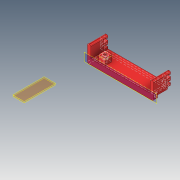
# Autodesk Inventor part: Prova A1
Saved by Autodesk Inventor 2019 (Build 230136000, 136)
## iProperties
Created: 2019-05-06
Part Number: Prova A1
Material: Generic
Document SubType Name: Modeling
Designer: giacomo
Density: 1 g/cm^3
Appearance: Light Red
Author: giacomo
Autodesk Inventor part; units mm, degrees
ref_plane "YZ Plane" through (0, 0, 0) normal (1, 0, 0) x (0, 1, 0)
ref_plane "XZ Plane" through (0, 0, 0) normal (0, 1, 0) x (-1, 0, 0)
ref_plane "XY Plane" through (0, 0, 0) normal (0, 0, 1) x (1, 0, 0)
sketch "Sketch1" plane through (0, 0, 0) normal (0, 1, 0) x (-1, 0, 0)
  line L0 (-50, 75) -> (50, 75)
  line L1 (50, 75) -> (50, -75)
  line L2 (50, -75) -> (-50, -75)
  line L3 (-50, -75) -> (-50, 75)
  line L4 (-50, 75) -> (50, -75) construction
  line L5 (50, 75) -> (-50, -75) construction
  point P0 (0, 0)
  dimension "d0" = 100
  dimension "d1" = 150
  constraints: 12 end point, 2 midpoint, 2 parallel, 1 horizontal, 1 perpendicular
  measures "d0" distance of L1.end L2.end
  measures "d1" distance of L0.end L1.end
extrude "Extrusion1" add sketch "Sketch1" along normal blind 8
sketch "Sketch3" plane through (0, 8, 0) normal (0, 1, 0) x (1, 0, 0)
  line L0 (-50, -75) -> (50, -75) projected
  line L1 (50, -75) -> (50, 75) projected
  line L2 (50, 75) -> (-50, 75) projected
  line L3 (-50, 75) -> (-50, -75) projected
  line L4 (45, 75) -> (45, -70)
  line L5 (-50, -75) -> (50, -75) projected
  line L6 (50, -75) -> (50, 75) projected
  line L7 (0, 0) -> (0, -83) construction
  line L8 (-45, 75) -> (-45, -70)
  line L9 (45, -70) -> (-45, -70)
  dimension "d4" = 5
  dimension "d5" = 5
  constraints: 8 end point, 3 parallel, 2 point on line, 1 perpendicular, 1 vertical, 1 other
  measures "d4" distance between parallel lines of L1 L4
  measures "d5" distance between parallel lines of L9 L0
extrude "Extrusion2" add sketch "Sketch3" along normal blind 18 contours L3 L2 L8 L9 L4 L1 L0
sketch "Sketch4" plane through (50, 0, -75) normal (0, 0, -1) x (-1, 0, 0)
  line L0 (100, 0) -> (0, 0) projected
  line L1 (100, 0) -> (100, 26) projected
  line L2 (95, 26) -> (100, 26) projected
  line L3 (95, 8) -> (95, 26) projected
  line L4 (5, 8) -> (95, 8) projected
  line L5 (5, 8) -> (5, 26) projected
  line L6 (0, 26) -> (5, 26) projected
  line L7 (0, 0) -> (0, 26) projected
  line L8 (95, 8) -> (5, 8) projected
  line L9 (5, 8) -> (5, 0)
  line L10 (95, 8) -> (95, 0)
  line L11 (0, 0) -> (100, 0) projected
  line L12 (0, 0) -> (0, 26) projected
  line L13 (5, 3) -> (95, 3)
  line L14 (5, 8) -> (95, 8) projected
  line L15 (5, 6) -> (95, 6)
  line L16 (5, 8) -> (0, 8)
  line L17 (100, 0) -> (0, 0) projected
  point P0 (50, 0)
  dimension "d8" = 3
  dimension "d9" = 3
  constraints: 10 end point, 8 point on line, 6 parallel, 2 perpendicular, 1 vertical
  measures "d8" distance between parallel lines of L0 L13
  measures "d9" distance between parallel lines of L13 L15
extrude "Extrusion3" add sketch "Sketch4" along normal blind 20 contours L0 L10 L3 L2 L1 | L0 L9 L13 L10 | L15 L9 L4 L10 | L7 L6 L5 L16
sketch "Sketch6" plane through (50, 0, 75) normal (1, 0, 0) x (0, 0, -1)
  line L0 (150, 0) -> (150, 8)
  line L1 (170, 26) -> (170, 8)
  line L2 (0, 0) -> (0, 26) projected
  line L3 (150, 8) -> (170, 8)
  line L4 (170, 26) -> (170, 8) projected
  line L5 (170, 11.2) -> (163, 9.7)
  line L6 (163, 9.7) -> (163, 15.7)
  line L7 (163, 15.7) -> (170, 14.2)
  line L8 (170, 19.3) -> (163, 17.8)
  line L9 (163, 17.8) -> (163, 23.8)
  line L10 (163, 23.8) -> (170, 22.3)
  line L11 (170, 22.3) -> (170, 19.3)
  line L12 (170, 14.2) -> (170, 11.2)
  point P0 (75, 0)
  dimension "d14" = 3
  dimension "d15" = 7
  dimension "d16" = 1.5
  dimension "d17" = 1.5
  dimension "d18" = 3
  dimension "d19" = 1.5
  dimension "d20" = 1.5
  dimension "d21" = 5.1
  dimension "d22" = 7
  dimension "d36" = 1.7
  constraints: 22 end point, 2 point on line, 2 vertical, 1 collinear, 1 horizontal, 1 parallel
  measures "d14" distance of L5.start L7.end
  measures "d15" distance between parallel lines of L1 L6
  measures "d16" vertical distance of L5.end L5.start
  measures "d17" vertical distance of L6.end L7.end
  measures "d18" distance of L8.start L10.end
  measures "d19" vertical distance of L8.end L8.start
  measures "d20" vertical distance of L10.start L10.end
  measures "d21" distance of L7.end L8.start
  measures "d22" distance between parallel lines of L4 L9
  measures "d36" distance from line of L3 L5.end
extrude "Extrusion4" cut sketch "Sketch6" against normal through all
fillet "Fillet1" radius 2 11 edges at (50, 0, 0) (50, 26, -10) (50, 13, 75) (0, 26, 75) (0, 0, 75) (-50, 26, -10) (-50, 13, 75) (-50, 0, -10) (45, 26, -12.5) (-45, 26, -12.5) (0, 26, 70)
sketch "Sketch11" plane through (-50, 9.7, -88) normal (-1, 0, 0) x (0, 0, 1)
  line L0 (9, 17.5) -> (0, 19.5) projected
  line L1 (0, 19.5) -> (0, 11.5) projected
  line L2 (0, 11.5) -> (9, 14) projected
  line L3 (9, 17.5) -> (9, 14) projected
  line L4 (9, 6) -> (0, 8.5) projected
  line L5 (0, 0) -> (9, 2.5) projected
  line L6 (0, 6) -> (0, 0) projected
  line L7 (9, 6) -> (9, 2.5) projected
  point P0 (88, -9.7)
sketch "Sketch12" plane through (-50, 2, 73) normal (-1, 0, 0) x (0, 0, 1)
  line L0 (-168, 28) -> (-168, 20)
  line L1 (-159, 26) -> (-168, 28)
  line L2 (-159, 26) -> (-159, 22.5)
  line L3 (-168, 20) -> (-159, 22.5)
  line L4 (-168, 17) -> (-168, 8.5)
  line L5 (-159, 14.5) -> (-168, 17)
  line L6 (-159, 14.5) -> (-159, 11)
  line L7 (-168, 8.5) -> (-159, 11)
  line L8 (-168, 0) -> (-168, 22) projected
  line L9 (-161, 19.2) -> (-161, 27.2) projected
  line L10 (-161, 27.2) -> (-168, 27.2)
  line L11 (-168, 22) -> (-168, 6) projected
  line L12 (-159, 17) -> (-168, 17)
  point P0 (-73, -2)
  constraints: 20 end point, 2 perpendicular, 2 point on line
sketch "Sketch15" plane through (45, 6, -75) normal (1, 0, 0) x (0, 0, -1)
  line L0 (0, 0) -> (0, 2) projected
  line L1 (0, 0) -> (20, 0) projected
  line L2 (20, 2) -> (20, 0) projected
  line L3 (0, 2) -> (20, 2) projected
  point P0 (-75, -6)
extrude "Extrusion8" add sketch "Sketch15" along normal blind 2.5
sketch "Sketch16" plane through (0, 8, 0) normal (0, 1, 0) x (1, 0, 0)
  line L0 (-45, -35) -> (-37, -35)
  line L1 (-37, -35) -> (-37, -15)
  line L2 (-37, -15) -> (-45, -15)
  line L3 (-45, -15) -> (-45, -35)
  line L4 (45, -70) -> (-45, -70) projected
  line L5 (-45, -70) -> (-45, 95) projected
  line L6 (32, -70) -> (45, -70)
  line L7 (45, -70) -> (45, -45)
  line L8 (45, -45) -> (32, -45)
  line L9 (32, -45) -> (32, -70)
  line L10 (45, 95) -> (45, -70) projected
  point P0 (0, 0)
  dimension "d39" = 35
  dimension "d40" = 0
  dimension "d41" = 8
  dimension "d42" = 20
  dimension "d43" = 0
  dimension "d44" = 0
  dimension "d45" = 25
  dimension "d46" = 13
  constraints: 16 end point, 4 parallel, 2 horizontal, 2 perpendicular
  measures "d39" distance between parallel lines of L4 L0
  measures "d40" distance between parallel lines of L5 L3
  measures "d41" distance between parallel lines of L1 L3
  measures "d42" distance of L0.end L1.end
  measures "d43" distance between parallel lines of L4 L6
  measures "d44" distance between parallel lines of L10 L7
  measures "d45" distance of L8.end L6.start
  measures "d46" distance of L7.end L8.end
extrude "Extrusion9" add sketch "Sketch16" along normal blind 16
fillet "Fillet4" radius 1 8 edges at (32, 24, 57.5) (38.5, 24, 45) (32, 16, 45) (-37, 24, 25) (-37, 16, 15) (-41, 24, 35) (-41, 24, 15) (-37, 16, 35)
sketch "Sketch17" plane through (0, 24, 0) normal (0, 1, 0) x (1, 0, 0)
  circle A0 centre (-41.5, -25) radius 2.1
  line L0 (-45, -34) -> (-45, -16) projected
  line L1 (-38, -34) -> (-45, -34) projected
  circle A1 centre (39, -58) radius 2.1
  line L2 (33, -70) -> (33, -46) projected
  line L3 (33, -46) -> (45, -46) projected
  point P0 (0, 0)
  dimension "d50" = 4.2
  dimension "d51" = 3.5
  dimension "d52" = 9
  dimension "d53" = 4.2
  dimension "d54" = 6
  dimension "d55" = 12
  constraints: 2 centre point
  measures "d50" diameter of A0
  measures "d51" distance from line of L0 A0.centre
  measures "d52" distance from line of L1 A0.centre
  measures "d53" diameter of A1
  measures "d54" distance from line of L2 A1.centre
  measures "d55" distance from line of L3 A1.centre
extrude "Extrusion10" cut sketch "Sketch17" against normal blind 8
sketch "Sketch18" plane through (-45, 9.7, -88) normal (1, 0, 0) x (0, 0, -1)
  circle A0 centre (-58, 11.3) radius 2.15
  circle A1 centre (-27.2, 11.3) radius 2.15
  line L0 (0, 8.1) -> (0, 14.1) projected
  line L1 (-27.2, 11.3) -> (-58, 11.3)
  line L2 (7, 16.3) -> (-160, 16.3) projected
  line L3 (-158, -1.7) -> (-158, 14.3) projected
  point P0 (-88, -9.7)
  dimension "d60" = 4.3
  dimension "d61" = 4.3
  dimension "d62" = 30.8
  dimension "d64" = 5
  dimension "d67" = 100
  constraints: 2 centre point, 2 end point, 1 horizontal
  measures "d60" diameter of A0
  measures "d61" diameter of A1
  measures "d62" distance of L1.start L1.end
  measures "d64" distance between parallel lines of L1 L2
  measures "d67" distance from line of L3 L1.end
extrude "Extrusion11" cut sketch "Sketch18" against normal through all
sketch "Sketch19" plane through (0, 24, 0) normal (0, 1, 0) x (1, 0, 0)
  circle A0 centre (-41.5, -25) radius 2.1 projected
  line L0 (-42, -22) -> (-39.1519, -23.067)
  line L1 (-39.1519, -23.067) -> (-38.6519, -26.067)
  line L2 (-38.6519, -26.067) -> (-41, -28)
  line L3 (-41, -28) -> (-43.8481, -26.933)
  line L4 (-43.8481, -26.933) -> (-44.3481, -23.933)
  line L5 (-44.3481, -23.933) -> (-42, -22)
  point P0 (0, 0)
  constraints: 12 end point, 2 coincident, 13 other
ref_plane "Work Plane2" through (0, 18, 0) normal (0, 1, 0) x (1, 0, 0)
ref_plane "Work Plane1" through (0, 20, 0) normal (0, 1, 0) x (1, 0, 0)
extrude "Extrusion12" cut sketch "Sketch19" against normal up to surface (2 mm away) from surface at -4
ref_plane "Work Plane3" through (50, 0, -69) normal (0, 0, -1) x (-1, 0, 0)
sketch "Sketch20" plane through (50, 0, -69) normal (0, 0, -1) x (-1, 0, 0)
  line L0 (-27, 40) -> (133, 40)
  line L1 (133, 40) -> (133, -17)
  line L2 (133, -17) -> (-27, -17)
  line L3 (-27, -17) -> (-27, 40)
  point P0 (50, 0)
  constraints: 8 end point, 2 parallel, 1 horizontal, 1 perpendicular
extrude "Extrusion13" cut sketch "Sketch20" against normal through all
sketch "Sketch21" plane through (0, 8, 0) normal (0, 1, 0) x (1, 0, 0)
  line L0 (-25, 71) -> (-35, 71)
  line L1 (-35, 71) -> (-35, 81)
  line L2 (-35, 81) -> (-25, 81)
  line L3 (-25, 81) -> (-25, 71)
  circle A0 centre (-30, 76) radius 2.1
  line L4 (-70, 69) -> (70, 69) projected
  line L5 (-45, 69) -> (-45, 95) projected
  point P0 (0, 0)
  dimension "d76" = 4.2
  dimension "d77" = 2
  dimension "d78" = 10
  dimension "d79" = 5
  dimension "d80" = 10
  dimension "d81" = 10
  dimension "d82" = 5
  constraints: 8 end point, 2 parallel, 1 centre point, 1 horizontal, 1 perpendicular
  measures "d76" diameter of A0
  measures "d77" distance between parallel lines of L4 L0
  measures "d78" distance between parallel lines of L2 L0
  measures "d79" distance from line of L0 A0.centre
  measures "d80" distance between parallel lines of L5 L1
  measures "d81" distance of L0.start L0.end
  measures "d82" distance from line of L1 A0.centre
extrude "Extrusion14" add sketch "Sketch21" along normal blind 10
ref_plane "Work Plane4" through (0, 16.5, 0) normal (0, 1, 0) x (1, 0, 0)
sketch "Sketch22" plane through (0, 16.5, 0) normal (0, 1, 0) x (1, 0, 0)
  line L0 (-32.0207, 72.5) -> (-34.0415, 76)
  line L1 (-34.0415, 76) -> (-32.0207, 79.5)
  line L2 (-32.0207, 79.5) -> (-27.9793, 79.5)
  line L3 (-27.9793, 79.5) -> (-25.9585, 76)
  line L4 (-25.9585, 76) -> (-27.9793, 72.5)
  line L5 (-27.9793, 72.5) -> (-32.0207, 72.5)
  point P0 (0, 0)
  point P1 (-30, 76)
  dimension "d88" = 7
  constraints: 12 end point, 13 other
  measures "d88" distance between parallel lines of L2 L5
extrude "Extrusion15" cut sketch "Sketch22" against normal blind 3.15
body "Solid1"
